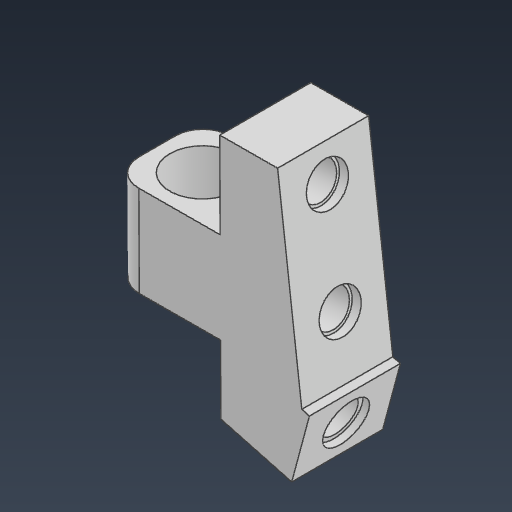
# Autodesk Inventor part: front-fight-holder
Saved by Autodesk Inventor 2023 (Build 270158000, 158)
## iProperties
Created: 2025-04-06
Part Number: front-fight-holder
Material: Generic
Document SubType Name: Modeling
Designer: szymo
Density: 1 g/cm^3
Appearance: Default
Mass: 2.71697 g
Surface Area: 19.8894 cm^2
Volume: 2.71697 cm^3
Author: szymo
Autodesk Inventor part; units mm, degrees
ref_plane "YZ Plane" through (0, 0, 0) normal (1, 0, 0) x (0, 1, 0)
ref_plane "XZ Plane" through (0, 0, 0) normal (0, 1, 0) x (-1, 0, 0)
ref_plane "XY Plane" through (0, 0, 0) normal (0, 0, 1) x (1, 0, 0)
sketch "Sketch1" plane through (0, 0, 0) normal (0, 0, 1) x (1, 0, 0)
  line L0 (-2.6739, 13.5718) -> (0.8124, -14.8221) projected
  line L1 (0.8124, -14.8221) -> (2.9187, -15.5653) projected
  line L2 (2.9187, -15.5653) -> (-0.66, 13.5807) projected
  line L3 (-0.66, 13.5807) -> (-2.6739, 13.5718) projected
  line L4 (-0.2713, -22.4751) -> (8.422, -24.8045) projected
  line L5 (8.422, -24.8045) -> (3.1187, -15.6189) projected
  line L6 (3.1187, -15.6189) -> (1.6698, -15.2307) projected
  line L7 (1.6698, -15.2307) -> (-0.2713, -22.4751) projected
  line L8 (0.2376, 6.2707) -> (1.0297, -0.1809)
  line L9 (0.2376, 6.2707) -> (-1.0249, 4.6548)
  line L10 (1.0297, -0.1809) -> (-0.5862, 1.0816)
  line L11 (-1.0249, 4.6548) -> (-8.0224, 3.7956)
  line L12 (-8.0224, 3.7956) -> (-7.5836, 0.2224)
  line L13 (-7.5836, 0.2224) -> (-0.5862, 1.0816)
  line L14 (-8.1686, 4.9867) -> (-7.4374, -0.9686)
  line L15 (-7.4374, -0.9686) -> (-2.4747, -0.3593)
  line L16 (-2.4747, -0.3593) -> (-3.2059, 5.596)
  line L17 (-3.2059, 5.596) -> (-8.1686, 4.9867)
  line L18 (1.6391, -5.1436) -> (2.4312, -11.5951)
  line L19 (1.6391, -5.1436) -> (0.3766, -6.7595)
  line L20 (2.4312, -11.5951) -> (0.8153, -10.3327)
  line L21 (0.3766, -6.7595) -> (-6.6209, -7.6187)
  line L22 (-6.6209, -7.6187) -> (-6.1821, -11.1918)
  line L23 (-6.1821, -11.1918) -> (0.8153, -10.3327)
  line L24 (-6.7671, -6.4276) -> (-6.0359, -12.3829)
  line L25 (-6.0359, -12.3829) -> (-1.0732, -11.7735)
  line L26 (-1.0732, -11.7735) -> (-1.8044, -5.8183)
  line L27 (-1.8044, -5.8183) -> (-6.7671, -6.4276)
  line L28 (2.4312, -11.5951) -> (2.9187, -15.5653) construction
  line L29 (1.6391, -5.1436) -> (1.0297, -0.1809) construction
  line L30 (-20.9088, -12.9407) -> (-20.9532, -2.9408)
  line L31 (-13.9089, -12.9096) -> (-13.9533, -2.9097)
  line L32 (-1.8394, -2.8559) -> (-8.8393, -2.887) projected
  line L33 (-21.3301, 2.0576) -> (-14.008, 2.0576)
  line L34 (-0.2713, -22.4751) -> (-8.0559, -20.3893)
  line L35 (-8.0559, -20.3893) -> (-8.1686, 4.9867)
  line L36 (-8.1686, 4.9867) -> (-8.1757, 6.574)
  line L37 (-88.1508, 17.361) -> (-90.1508, 17.3522) projected
  line L38 (-8.1757, 6.574) -> (-1.8182, 6.6022)
  line L39 (0.8124, -14.8221) -> (0.8351, -15.007)
  line L40 (0.8351, -15.007) -> (1.6698, -15.2307)
  line L41 (-9.0157, -12.8878) -> (-8.9913, -18.3878) projected
  point P0 (0, 0)
  dimension "d0" = 6.5
  dimension "d2" = 3.6
  dimension "d3" = 8.5
  dimension "d7" = 45
  dimension "d9" = 6
  dimension "d10" = 1.2
  dimension "d11" = 1.2
  dimension "d12" = 5
  dimension "d13" = 6.5
  dimension "d14" = 3.6
  dimension "d15" = 8.5
  dimension "d16" = 45
  dimension "d17" = 6
  dimension "d18" = 1.2
  dimension "d19" = 1.2
  dimension "d20" = 5
  dimension "d21" = 4
  dimension "d22" = 5
  dimension "d23" = 5
  dimension "d43" = 1
  constraints: 62 end point, 14 perpendicular, 7 collinear, 6 parallel, 6 point on line, 1 horizontal, 6 other
  measures "d0" distance of L8.start L8.end
  measures "d2" distance of L11.end L12.end
  measures "d3" distance between parallel lines of L12 L8
  measures "d7" angle of L8 L9
  measures "d9" distance between parallel lines of L15 L17
  measures "d10" distance between parallel lines of L11 L17
  measures "d11" distance between parallel lines of L15 L13
  measures "d12" distance of L14.end L15.end
  measures "d13" distance of L19.start L18.end
  measures "d14" distance of L21.end L23.start
  measures "d15" distance between parallel lines of L22 L18
  measures "d16" angle of L18 L19
  measures "d17" distance between parallel lines of L25 L27
  measures "d18" distance between parallel lines of L21 L27
  measures "d19" distance between parallel lines of L25 L23
  measures "d20" distance of L24.end L25.end
  measures "d21" distance of L1.end L18.end
  measures "d22" distance of L8.end L19.start
  measures "d23" distance from line of L32 L33.start
  measures "d43" distance from line of L38 L16.end
extrude "Extrusion1" add sketch "Sketch1" against normal blind 10 contours L0 L11 L16 L17 L36 L38 | L0 L13 L16 L11 | L0 L21 L26 L27 L24 L22 L25 L23 L39 L40 L7 L34 L35 L14 L12 L15 L16 L13 | L16 L13 L12 L11 | L11 L14 L17 L16 | L0 L23 L26 L21 | L16 L15 L14 L13 | L26 L23 L22 L21 | L21 L24 L27 L26 | L26 L25 L24 L23
sketch "Sketch2" plane through (0.8351, -15.007, 0) normal (0.9925462, 0.1218693, 0) x (0, 0, -1)
  line L0 (0, 21.1919) -> (0, 19.7419) projected
  line L1 (0, 14.6919) -> (0, 16.1419) projected
  line L2 (0, 9.6919) -> (0, 8.2419) projected
  line L3 (0, 3.1919) -> (0, 4.6419) projected
  line L4 (10, 21.7715) -> (10, 0) projected
  line L5 (10, 21.1919) -> (0, 21.1919)
  line L6 (10, 14.6919) -> (0, 14.6919)
  line L7 (10, 3.1919) -> (0, 3.1919)
  line L8 (10, 9.6919) -> (0, 9.6919)
  line L9 (10, 3.1919) -> (0, 9.6919)
  line L10 (10, 9.6919) -> (0, 3.1919)
  line L11 (0, 14.6919) -> (10, 21.1919)
  line L12 (10, 14.6919) -> (0, 21.1919)
  point P0 (5, 17.9419)
  point P1 (5, 6.4419)
  constraints: 16 end point, 4 parallel, 4 point on line, 3 midpoint, 1 perpendicular
hole "Hole1" at (-1.3515, 2.8012, -5) at (0.05, -8.6131, -5) direction (-0.9925462, -0.1218693, 0) diameter 4 depth 6 counterbore diameter 4.6 counterbore depth 1
ref_plane "Work Plane1" through (-48.5153, -13.0633, -49.5) normal (-0.0044406, 0.9999901, 0) x (-0.9999901, -0.0044406, 0)
sketch "Sketch3" plane through (-48.5153, -13.0633, -49.5) normal (-0.0044406, 0.9999901, 0) x (-0.9999901, -0.0044406, 0)
  circle A0 centre (-33.5, 44.5) radius 3.5 projected
  line L0 (-46.784, 49.5) -> (-40.4265, 49.5) projected
  line L1 (-46.784, 49.5) -> (-46.784, 39.5) projected
  line L2 (-40.4265, 39.5) -> (-46.784, 39.5) projected
  line L3 (-40.4265, 49.5) -> (-40.4265, 39.5) projected
  line L4 (-40.4265, 49.5) -> (-40.4265, 39.5) projected
  line L5 (-40.4265, 39.5) -> (-28.5, 39.5)
  line L6 (-28.5, 39.5) -> (-28.5, 49.5)
  line L7 (-28.5, 49.5) -> (-40.4265, 49.5)
  line L8 (-33.5, 44.5) -> (-30, 44.5)
  circle A1 centre (-33.5, 44.5) radius 3.6
  point P0 (-48.5728, 49.5)
  point P1 (-33.5, 41)
  point P2 (-33.5, 48)
  point P3 (-28.5, 44.5)
  dimension "d36" = 1.5
  dimension "d37" = 1.5
  dimension "d38" = 1.5
  dimension "d39" = 7.2
  constraints: 8 end point, 3 point on circle, 2 horizontal, 2 perpendicular, 1 centre point, 1 coincident, 1 midpoint
  measures "d36" distance from line of L5 A0.start
  measures "d37" distance from line of L7 A0.end
  measures "d38" distance of point (-28.5, 44.5) L8.end
  measures "d39" diameter of A1
ref_plane "Work Plane2" through (-17.5011, -2.9254, -9.9411) normal (-0.0044406, 0.9999901, 0) x (0.6640065, 0.0029486, 0.747721)
extrude "Extrusion2" add sketch "Sketch3" along normal up to surface (10 mm away) contours L7 L6 L5 L3
fillet "Fillet1" radius 3 2 edges at (-20.0378, -7.9367, 0) (-20.0378, -7.9367, -10)
sketch "Sketch4" plane through (-0.2713, -22.4751, 0) normal (0.9659258, -0.258819, 0) x (0, 0, -1)
  circle A0 centre (5, 3.75) radius 1.6 projected
  point P0 (0, 21.7795)
  constraints: 1 coincident
hole "Hole2" at (0.6992, -18.8529, -5) direction (-0.9659258, 0.258819, 0) diameter 4 depth 5 counterbore diameter 5 counterbore depth 0.75
sketch "Sketch5" plane through (-4.1304, -17.5588, -5) normal (0.9659258, -0.258819, 0) x (0, 0, -1)
  circle A0 centre (0, 0) radius 1.6 projected
  circle A1 centre (0, 0) radius 2 projected
  point P0 (-5, 18.0295)
  constraints: 1 coincident
hole "Hole3" at (-4.1304, -17.5588, -5) direction (-0.9659258, 0.258819, 0) diameter 2.8 depth 5 countersink diameter 3.9 countersink angle 90
equation "\"d10\" = d11"
equation "\"d18\" = d19"
body "Solid1"
